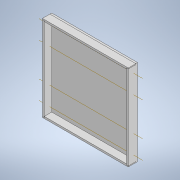
# Autodesk Inventor part: Bottom Base
Saved by Autodesk Inventor 2022 (Build 260153000, 153)
## iProperties
Created: 2022-04-03
Part Number: Bottom Base
Material: Generic
Document SubType Name: Modeling
Designer: Nick
Density: 1 g/cm^3
Appearance: Default
Author: Nick
Autodesk Inventor part; units mm, degrees
ref_plane "YZ Plane" through (0, 0, 0) normal (1, 0, 0) x (0, 1, 0)
ref_plane "XZ Plane" through (0, 0, 0) normal (0, 1, 0) x (-1, 0, 0)
ref_plane "XY Plane" through (0, 0, 0) normal (0, 0, 1) x (1, 0, 0)
sketch "Sketch1" plane through (0, 0, 0) normal (0, 0, 1) x (1, 0, 0)
  line L0 (0, 0) -> (292.1, 0)
  line L1 (292.1, 0) -> (292.1, 292.1)
  line L2 (292.1, 292.1) -> (0, 292.1)
  line L3 (0, 292.1) -> (0, 0)
  dimension "d11" = 292.1
  dimension "d12" = 292.1
  constraints: 8 end point, 2 parallel, 1 horizontal, 1 perpendicular
  measures "d11" distance of L2.end L1.end
  measures "d12" distance of L1.end L0.end
extrude "Extrusion3" add sketch "Sketch1" along normal blind 31.75
sketch "Sketch2" plane through (0, 0, 0) normal (-1, 0, 0) x (0, 0, 1)
  line L0 (31.75, 0) -> (31.75, 292.1) projected
  line L1 (31.75, 0) -> (31.75, 88.9)
  line L2 (31.75, 292.1) -> (31.75, 203.2)
  point P0 (0, 0)
  dimension "d15" = 88.9
  dimension "d16" = 88.9
  constraints: 4 end point, 2 coincident, 2 point on line
  measures "d15" distance of L0.start L1.end
  measures "d16" distance of L0.end L2.end
shell "Shell1" thickness 6.35 removed faces 1 at (97.3667, 194.7333, 31.75)
sketch "Sketch3" plane through (6.35, 6.35, 6.35) normal (1, 0, 0) x (0, 0, -1)
  line L0 (0, 279.4) -> (0, 0) projected
  line L1 (0, 279.4) -> (-25.4, 279.4) projected
  line L2 (-25.4, 0) -> (-25.4, 279.4) projected
  line L3 (0, 0) -> (-25.4, 0) projected
  line L4 (0, 279.4) -> (-25.4, 279.4) projected
  line L5 (-25.4, 260.35) -> (0, 260.35) construction
  line L6 (0, 279.4) -> (0, 0) projected
  line L7 (6.35, 285.75) -> (-25.4, 285.75) projected
  line L8 (6.35, -6.35) -> (-25.4, -6.35) projected
  point P0 (-6.5, 260.35)
  point P1 (-6.5, 196.85)
  point P2 (-6.5, 82.55)
  point P3 (-6.5, 19.05)
  dimension "d20" = 25.4
  dimension "d22" = 88.9
  dimension "d23" = 88.9
  dimension "d24" = 25.4
  dimension "d28" = 6.5
  constraints: 3 point on line, 3 vertical alignment, 2 end point, 1 perpendicular
  measures "d20" distance between parallel lines of L5 L7
  measures "d22" distance from line of L7 point (-6.5, 196.85)
  measures "d23" distance from line of L8 point (-6.5, 82.55)
  measures "d24" distance from line of L8 point (-6.5, 19.05)
  measures "d28" distance from line of L0 point (-6.5, 260.35)
sketch "Sketch6" plane through (0, 0, 31.75) normal (0, 0, 1) x (1, 0, 0)
  line L0 (285.75, 6.35) -> (6.35, 6.35) projected
  line L1 (6.35, 6.35) -> (6.35, 285.75) projected
  line L2 (6.35, 285.75) -> (285.75, 285.75) projected
  line L3 (285.75, 285.75) -> (285.75, 6.35) projected
  line L4 (292.1, 0) -> (292.1, 292.1) projected
  line L5 (292.1, 292.1) -> (0, 292.1) projected
  line L6 (0, 292.1) -> (0, 0) projected
  line L7 (0, 0) -> (292.1, 0) projected
  line L8 (6.35, 285.75) -> (6.35, 6.35) projected
  line L9 (6.35, 6.35) -> (6.35, 3.175)
  line L10 (6.35, 3.175) -> (0, 3.175)
  line L11 (0, 292.1) -> (0, 0) projected
  line L12 (0, 6.35) -> (0, 0)
  line L13 (292.1, 0) -> (292.1, 292.1) projected
  line L14 (292.1, 0) -> (292.1, 6.35)
  line L15 (6.35, 6.35) -> (285.75, 6.35) projected
  line L16 (285.75, 6.35) -> (285.75, 3.175)
  line L17 (285.75, 3.175) -> (292.1, 3.175)
  line L18 (0, 292.1) -> (0, 285.75)
  line L19 (6.35, 285.75) -> (6.35, 288.925)
  line L20 (6.35, 288.925) -> (0, 288.925)
  line L21 (6.35, 285.75) -> (285.75, 285.75) projected
  line L22 (285.75, 285.75) -> (285.75, 288.925)
  line L23 (285.75, 288.925) -> (292.1, 288.925)
  line L24 (292.1, 292.1) -> (292.1, 285.75)
  point P0 (0, 3.175)
  point P1 (0, 288.925)
  constraints: 24 end point, 7 point on line, 4 midpoint, 4 vertical, 3 horizontal alignment, 2 horizontal, 2 perpendicular, 1 collinear
extrude "Extrusion6" add sketch "Sketch6" against normal up to surface (25.4 mm away) separate body contours L16 L17 L4 L7 L6 L10 L9 L0
extrude "Extrusion7" add sketch "Sketch6" against normal up to surface (25.4 mm away) separate body contours L2 L19 L20 L6 L5 L4 L23 L22
combine bodies "Combine1" operation type subtract main body 1 bodies to subtract 3 keep tools yes
combine bodies "Combine2" operation type subtract main body 1 bodies to subtract 2 keep tools yes
sketch "Sketch4" plane through (285.75, 6.35, 6.35) normal (-1, 0, 0) x (0, 0, 1)
  line L0 (0, 0) -> (0, 279.4) projected
  line L1 (0, 0) -> (19.05, 0) projected
  line L2 (19.05, 279.4) -> (19.05, 0) projected
  line L3 (0, 279.4) -> (19.05, 279.4) projected
  line L4 (19.05, 0) -> (0, 21.4113)
  line L5 (0, 0) -> (0, 279.4) projected
  point P0 (-6.35, -6.35)
  point P1 (0, 21.4113)
  dimension "d25" = 41.66
  constraints: 2 end point, 1 point on line
  measures "d25" angle of L4 L0
equation "\"d23\" = d22"
equation "\"d24\" = d20"
body "Solid2"
body "Solid3"
body "Solid4"
